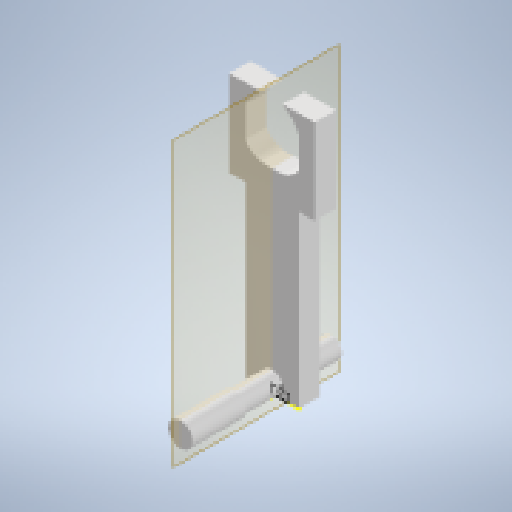
# Autodesk Inventor part: brazo2
Saved by Autodesk Inventor 2023 (Build 270158000, 158)
## iProperties
Created: 2024-08-03
Part Number: brazo2
Material: Generic
Document SubType Name: Modeling
Designer: sebas
Density: 1 g/cm^3
Appearance: Default
Mass: 27.7155 g
Surface Area: 86.0835 cm^2
Volume: 27.7155 cm^3
Author: sebas
Autodesk Inventor part; units mm, degrees
ref_plane "YZ Plane" through (0, 0, 0) normal (1, 0, 0) x (0, 1, 0)
ref_plane "XZ Plane" through (0, 0, 0) normal (0, 1, 0) x (-1, 0, 0)
ref_plane "XY Plane" through (0, 0, 0) normal (0, 0, 1) x (1, 0, 0)
sketch "Sketch1" plane through (0, 0, 0) normal (0, 1, 0) x (-1, 0, 0)
  line L0 (0, 0) -> (0, -10)
  line L1 (0, 0) -> (25, 0)
  line L2 (25, 0) -> (25, -10)
  line L3 (25, -10) -> (0, -10)
  dimension "d0" = 10
  dimension "d1" = 25
  dimension "d2" = 10
  constraints: 8 end point, 1 horizontal, 1 perpendicular, 1 vertical
  measures "d0" distance of L0.start L0.end
  measures "d1" distance of L0.start L1.end
  measures "d2" distance of L1.end L2.end
extrude "Extrusion1" add sketch "Sketch1" along normal blind 120
sketch "Sketch2" plane through (-25, 0, 0) normal (0, 0, 1) x (1, 0, 0)
  line L0 (25, 0) -> (0, 0) projected
  line L1 (12.5, 0) -> (17.5, 0)
  line L2 (17.5, 0) -> (12.5, 0)
  line L3 (12.5, 0) -> (12.5, 4.9)
  circle A0 centre (12.5, 4.9) radius 4.9
  dimension "d5" = 5
  dimension "d6" = 4.9
  constraints: 6 end point, 1 coincident, 1 collinear, 1 midpoint, 1 perpendicular, 1 point on line, 1 vertical alignment, 2 other
  measures "d5" distance of L1.start L1.end
  measures "d6" distance of L1.start L3.end
extrude "Extrusion2" add sketch "Sketch2" along normal blind 18
sketch "Sketch3" plane through (-25, 120, 0) normal (0, 0, 1) x (1, 0, 0)
  line L0 (12.5, -120) -> (20.5, -120)
  line L1 (12.5, -120) -> (25, -120) projected
  dimension "d9" = 8
  constraints: 2 end point, 1 point on line
  measures "d9" distance of L0.start L0.end
sketch "Sketch4" plane through (0, 0, 0) normal (1, 0, 0) x (0, 0, -1)
  point P0 (0, 0)
sketch "Sketch5" plane through (0, 0, 0) normal (1, 0, 0) x (0, 0, -1)
  point P0 (0, 0)
sketch "Sketch6" plane through (0, 0, 0) normal (1, 0, 0) x (0, 0, -1)
  point P0 (0, 0)
sketch "Sketch7" plane through (0, 0, 0) normal (1, 0, 0) x (0, 0, -1)
  point P0 (0, 0)
sketch "Sketch8" plane through (0, 0, -10) normal (0, 0, -1) x (-1, 0, 0)
  circle A0 centre (12.5, 4.9) radius 4.9 projected
  circle A1 centre (12.5, 4.9) radius 4.9
  point P0 (0, 0)
  point P1 (12.5, 0)
  constraints: 2 vertical alignment, 1 coincident, 2 other
extrude "Extrusion3" add sketch "Sketch8" along normal blind 18
sketch "Sketch9" plane through (-12.5, 4.9, 18) normal (0, 0, 1) x (1, 0, 0)
  circle A0 centre (0, 0) radius 5.75
  point P0 (12.5, -4.9)
  dimension "d12" = 11.5
  constraints: 1 centre point
  measures "d12" diameter of A0
extrude "Extrusion4" add sketch "Sketch9" along normal blind 25
sketch "Sketch10" plane through (-25, 120, 0) normal (0, 0, 1) x (1, 0, 0)
  line L0 (0, 0) -> (25, 0) projected
  line L1 (12.5, 0) -> (12.5, -28.5)
  line L2 (12.5, -28.5) -> (-0.5, -28.5)
  line L3 (-0.5, -28.5) -> (12.5, -28.5)
  line L4 (12.5, -28.5) -> (25.5, -28.5)
  line L5 (25.5, -28.5) -> (25.5, 0)
  line L6 (25.5, 0) -> (-0.5, 0)
  line L7 (-0.5, 0) -> (-0.5, -28.5)
  line L8 (12.5, 0) -> (7.5, 0)
  line L9 (7.5, 0) -> (17.5, 0)
  line L10 (25.5, 0) -> (25.5, -10)
  line L11 (25.5, -10) -> (25.5, -22)
  line L12 (-0.5, 0) -> (-0.5, -10)
  line L13 (-0.5, -10) -> (-0.5, -22)
  arc A0 (7.5, 0) -> (-0.5, -22) centre (17.25, -16) ccw
  arc A1 (-0.5, -22) -> (12.5, -28.5) centre (10, -17.25) ccw
  line L14 (7.5, 0) -> (12.5, 0)
  arc A2 (25.5, -22) -> (17.5, 0) centre (7.75, -16) ccw
  arc A3 (12.5, -28.5) -> (25.5, -22) centre (15, -17.25) ccw
  line L15 (7.5, 0) -> (-7.5, 0)
  line L16 (-7.5, 0) -> (-7.5, -34)
  line L17 (-7.5, -34) -> (25, -34)
  line L18 (25, -120) -> (25, 0) projected
  line L19 (25, -34) -> (32.5, -34)
  line L20 (32.5, 0) -> (25, 0)
  line L21 (25, 0) -> (17.5, 0)
  line L22 (17.5, 0) -> (32.5, 0)
  line L23 (32.5, 0) -> (32.5, -34)
  point P0 (7.5, -28.5)
  point P1 (17.5, -28.5)
  point P2 (25, -22.9782)
  point P3 (25, -8.6856)
  dimension "d15" = 28.5
  dimension "d16" = 13
  dimension "d17" = 13
  dimension "d18" = 13
  dimension "d19" = 5
  dimension "d20" = 10
  dimension "d21" = 10
  dimension "d22" = 12
  dimension "d23" = 10
  dimension "d24" = 12
  dimension "d25" = 15
  dimension "d26" = 34
  dimension "d28" = 15
  constraints: 44 end point, 10 point on circle, 9 point on line, 5 perpendicular, 4 centre point, 3 collinear, 1 midpoint, 1 parallel, 1 vertical
  measures "d15" distance of L1.start L1.end
  measures "d16" distance of L1.end L2.end
  measures "d17" distance of L2.end L1.end
  measures "d18" distance of L1.end L4.end
  measures "d19" distance of L1.start L8.end
  measures "d20" distance of L8.end L9.end
  measures "d21" distance of L5.end L10.end
  measures "d22" distance of L10.end L11.end
  measures "d23" distance of L6.end L12.end
  measures "d24" distance of L12.end L13.end
  measures "d25" distance of L8.end L15.end
  measures "d26" distance of L15.end L16.end
  measures "d28" distance of L20.start L9.end
extrude "Extrusion5" cut sketch "Sketch10" against normal blind 10 contours L0 L1 L2 A1 L7 A0 | L0 A2 L18 A3 L4 L1
sketch "Sketch11" plane through (-25, 0, 0) normal (0, 0, 1) x (1, 0, 0)
  point P0 (25, 0)
sketch "Sketch12" plane through (-7.5, 120, 0) normal (0, 0, 1) x (1, 0, 0)
  line L0 (7.5, 0) -> (0, 0) projected
  line L1 (0, 0) -> (15, 0)
  line L2 (15, 0) -> (15, -40)
  line L3 (15, -40) -> (7.5, -40)
  line L4 (7.5, -120) -> (7.5, -22.9782) projected
  line L5 (7.5, -8.6856) -> (7.5, 0) projected
  line L6 (7.5, -40) -> (7.5, 0)
  line L7 (-10, 0) -> (-17.5, 0) projected
  line L8 (7.5, 0) -> (-17.5, 0)
  line L9 (-10, 0) -> (-25, 0)
  line L10 (-25, 0) -> (-25, -40.3744)
  line L11 (-25, -40.3744) -> (-17.5, -40.3744)
  line L12 (-17.5, -120) -> (-17.5, -22.9782) projected
  line L13 (-17.5, -8.6856) -> (-17.5, 0) projected
  line L14 (-17.5, -40.3744) -> (-17.5, 0)
  dimension "d31" = 15
  dimension "d32" = 40
  dimension "d33" = 15
  constraints: 18 end point, 4 perpendicular, 2 horizontal, 2 point on line, 2 vertical, 1 collinear
  measures "d31" distance of L0.end L1.end
  measures "d32" distance of L1.end L2.end
  measures "d33" distance of L7.start L9.end
extrude "Extrusion6" add sketch "Sketch12" against normal blind 10
ref_plane "Work Plane1" through (-12.5, 0, 0) normal (1, 0, 0) x (0, 0, -1)
body "Solid1"
